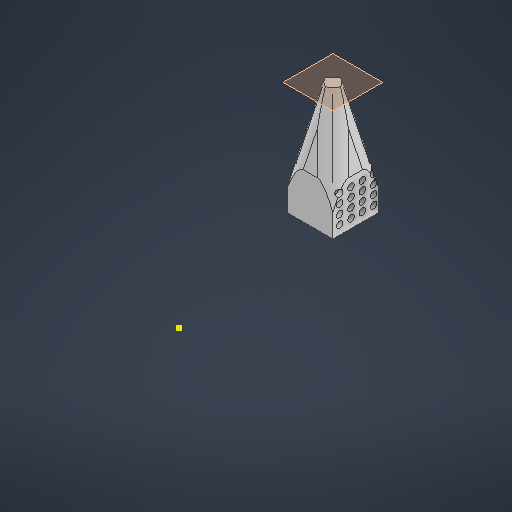
# Autodesk Inventor part: Part1
Saved by Autodesk Inventor 2025.1 (Build 291241000, 241)
## iProperties
Created: 2025-01-31
Part Number: Part1
Material: Generic
Document SubType Name: Modeling
Designer: Shane
Density: 1 g/cm^3
Appearance: Default
Author: Shane
Autodesk Inventor part; units mm, degrees
ref_plane "YZ Plane" through (0, 0, 0) normal (1, 0, 0) x (0, 1, 0)
ref_plane "XZ Plane" through (0, 0, 0) normal (0, 1, 0) x (-1, 0, 0)
ref_plane "XY Plane" through (0, 0, 0) normal (0, 0, 1) x (1, 0, 0)
sketch "Sketch1" plane through (0, 0, 0) normal (0, 1, 0) x (-1, 0, 0)
  line L0 (35, -59) -> (25, -59)
  line L1 (25, -59) -> (25, -69)
  line L2 (25, -69) -> (35, -69)
  line L3 (35, -69) -> (35, -59)
  dimension "d2" = 10
  dimension "d3" = 10
  constraints: 8 end point, 2 parallel, 1 horizontal, 1 perpendicular
  measures "d2" distance of L2.end L0.start
  measures "d3" distance of L1.end L2.end
extrude "Extrusion1" add sketch "Sketch1" along normal blind 10
ref_plane "Work Plane1" through (0, 25, 0) normal (0, 1, 0) x (1, 0, 0)
sketch "Sketch2" plane through (0, 25, 0) normal (0, 1, 0) x (1, 0, 0)
  point P0 (0, 0)
sketch "Sketch3" plane through (0, 25, 0) normal (0, 1, 0) x (1, 0, 0)
  line L0 (-25, 59) -> (-25, 69) construction
  line L1 (-25, 69) -> (-35, 69) construction
  line L2 (-35, 69) -> (-35, 59) construction
  line L3 (-35, 59) -> (-25, 59) construction
  line L4 (-32, 62) -> (-32, 66)
  line L5 (-32, 66) -> (-28, 66)
  line L6 (-28, 66) -> (-28, 62)
  line L7 (-28, 62) -> (-32, 62)
  point P0 (0, 0)
  constraints: 8 end point, 3 other
loft "Loft1" add profiles "Sketch3" section 1 edges at (-25, 10, -64) (-30, 10, -69) (-35, 10, -64) (-30, 10, -59)
shell "Shell1" thickness 1 removed faces 1 at (-28.3333, 0, -62.3333)
sketch "Sketch4" plane through (-25, 0, -59) normal (1, 0, 0) x (0, 0, -1)
  circle A0 centre (9, 8) radius 0.7097
  line L0 (10, 9.8251) -> (10, 0.5541) construction
  line L1 (10, 0) -> (10, 10) projected
  line L2 (10, 10) -> (1.3312, 10) construction
  line L3 (10, 10) -> (0, 10) projected
  line L4 (10, 10) -> (10, 6.2491)
  line L5 (10, 10) -> (6.0882, 10)
  circle A1 centre (6.5, 8) radius 0.7097
  circle A2 centre (4, 8) radius 0.7097
  circle A3 centre (1.5, 8) radius 0.7097
  circle A4 centre (9, 6) radius 0.7097
  circle A5 centre (6.5, 6) radius 0.7097
  circle A6 centre (4, 6) radius 0.7097
  circle A7 centre (1.5, 6) radius 0.7097
  circle A8 centre (9, 4) radius 0.7097
  circle A9 centre (6.5, 4) radius 0.7097
  circle A10 centre (4, 4) radius 0.7097
  circle A11 centre (1.5, 4) radius 0.7097
  circle A12 centre (9, 2) radius 0.7097
  circle A13 centre (6.5, 2) radius 0.7097
  circle A14 centre (4, 2) radius 0.7097
  circle A15 centre (1.5, 2) radius 0.7097
  point P0 (-59, 0)
  dimension "d12" = 2.5
  dimension "d15" = 2
  constraints: 16 centre point, 8 end point, 4 point on line, 1 horizontal, 1 vertical, 30 other
  measures "d12" distance of A0.centre A1.centre
  measures "d15" distance of A0.centre A4.centre
extrude "Extrusion2" cut sketch "Sketch4" against normal blind 2.75
fillet "Fillet1" radius 3.5 4 edges at (-26.5, 17.5, -60.5) (-26.5, 17.5, -67.5) (-33.5, 17.5, -60.5) (-33.5, 17.5, -67.5)
body "Solid1"
